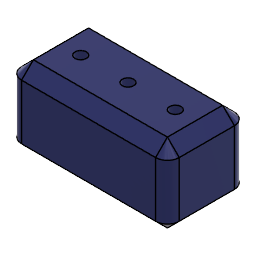
Bed Clamp (Autodesk Fusion 360 design; units mm, degrees)
Autodesk Fusion 360 part; units mm, degrees
sketch "Sketch1" plane through (0, 0, 0) normal (0, 1, 0) x (1, 0, 0)
  line L0 (0, 0) -> (40, 0)
  line L1 (40, 0) -> (40, 20)
  line L2 (40, 20) -> (0, 20)
  line L3 (0, 20) -> (0, 0)
  circle A0 centre (8, 10) radius 2.05
  circle A1 centre (20, 10) radius 2.05
  circle A2 centre (32, 10) radius 2.05
  circle A3 centre (8, 10) radius 2.8 construction
  circle A4 centre (32, 10) radius 2.8 construction
  line L4 (5.2, 8.3834) -> (8, 6.7668)
  line L5 (8, 6.7668) -> (10.8, 8.3834)
  line L6 (10.8, 8.3834) -> (10.8, 11.6166)
  line L7 (10.8, 11.6166) -> (8, 13.2332) construction
  line L8 (8, 13.2332) -> (5.2, 11.6166) construction
  line L9 (5.2, 11.6166) -> (5.2, 8.3834)
  line L10 (29.2, 8.3834) -> (32, 6.7668)
  line L11 (32, 6.7668) -> (34.8, 8.3834)
  line L12 (34.8, 8.3834) -> (34.8, 11.6166)
  line L13 (34.8, 11.6166) -> (32, 13.2332) construction
  line L14 (32, 13.2332) -> (29.2, 11.6166) construction
  line L15 (29.2, 11.6166) -> (29.2, 8.3834)
  line L16 (10.8, 11.6166) -> (10.8, 20)
  line L17 (5.2, 11.6166) -> (5.2, 20)
  line L18 (34.8, 11.6166) -> (34.8, 20)
  line L19 (29.2, 11.6166) -> (29.2, 20)
  circle A5 centre (20, 10) radius 1.45
  circle A6 centre (32, 10) radius 1.45
  circle A7 centre (8, 10) radius 1.45
  line L20 (17.2, 8.3834) -> (20, 6.7668)
  line L21 (20, 6.7668) -> (22.8, 8.3834)
  line L22 (22.8, 8.3834) -> (22.8, 11.6166)
  line L23 (22.8, 11.6166) -> (20, 13.2332) construction
  line L24 (20, 13.2332) -> (17.2, 11.6166) construction
  line L25 (17.2, 11.6166) -> (17.2, 8.3834)
  line L26 (17.2, 11.6166) -> (17.2, 20)
  line L27 (22.8, 11.6166) -> (22.8, 20)
  point P0 (8, 10)
  point P1 (32, 10)
  point P2 (20, 10)
  dimension "ClampWidth" = 20
  dimension "ClampLength" = 40
  dimension "MagnetHoleDia" = 4.1
  dimension "d7" = 10
  dimension "d11" = 8
  dimension "d14" = 24
  dimension "d15" = 0
  dimension "NutCircum" = 5.6
  dimension "d17" = 10
  dimension "d19" = 5.6
  dimension "d20" = 8
  dimension "d21" = 10
  dimension "d22" = 2.9
  dimension "ScrewDia" = 2.9
  dimension "d24" = 2.9
  constraint coincident L0.start L3.end
  constraint horizontal L0
  constraint perpendicular L0 L1
  constraint perpendicular L0 L3
  constraint horizontal L2
  constraint concentric A0 A3
  constraint coincident P0 A0.centre
  constraint coincident P1 A2.centre
  constraint tangent A3 L7
  constraint tangent A4 L14
  constraint vertical L9
  constraint vertical L12
  constraint coincident L2 L16.end
  constraint perpendicular L2 L16
  constraint coincident L2 L17.end
  constraint perpendicular L2 L17
  constraint coincident L2 L18.end
  constraint perpendicular L2 L18
  constraint coincident L2 L19.end
  constraint perpendicular L2 L19
  constraint concentric A1 A5
  constraint concentric A4 A6
  constraint concentric A0 A7
  constraint coincident P2 A1.centre
  constraint coincident L2 L26.end
  constraint perpendicular L2 L26
  constraint coincident L2 L27.end
  constraint perpendicular L2 L27
  constraint equal L6 L22
  constraint equal L16 L27
  measures "ClampWidth" distance of L0.end L1.end
  measures "ClampLength" distance of L0.start L0.end
  measures "MagnetHoleDia" diameter of A0
  measures "d7" distance of L0 P0
  measures "d11" distance of L3 P0
  measures "NutCircum" diameter of A3
  measures "d17" distance of L0 P0
  measures "d19" diameter of A4
  measures "d20" distance of L1 P1
  measures "d21" distance of L0 P1
  measures "d22" diameter of A5
  measures "ScrewDia" diameter of A6
  measures "d24" diameter of A7
extrude "Extrude1" add sketch "Sketch1" along normal blind 20 contours L0 L1 L2 L3 L4 L5 L6 L9 L10 L11 L12 L15 L16 L17 L18 L19 L20 L21 L22 L25 L26 L27 | L2 L4 L5 L6 L9 L16 L17 | L2 L10 L11 L12 L15 L18 L19 | L2 L20 L21 L22 L25 L26 L27 | A0 | A1 | A2 | A5 | A6 | A7
extrude "Extrude2" cut sketch "Sketch1" along normal blind 2.2 contours A0 | A1 | A2 | A5 | A6 | A7
extrude "Extrude3" cut sketch "Sketch1" along normal blind 20 contours A5 | A6 | A7
extrude "Extrude4" cut sketch "Sketch1" against normal blind 2.6 from surface at 15 contours L2 L4 L5 L6 L9 L16 L17 | L2 L10 L11 L12 L15 L18 L19 | L2 L20 L21 L22 L25 L26 L27 | A0 | A1 | A2
fillet "Fillet1" radius 3 4 edges at (40, 10, -20) (40, 10, 0) (0, 10, 0) (0, 10, -20)
chamfer "Chamfer1" distance 3 angle 45 8 edges at (20, 20, -20) (40, 20, -10) (20, 20, 0) (0, 20, -10) (0, 0, -10) (20, 0, -20) (20, 0, 0) (40, 0, -10)
equation "d7 = ClampWidth / 2"
equation "d11 = ClampLength / 5"
equation "d14 = ClampLength * 3 / 5"
equation "d17 = ClampWidth / 2"
equation "d19 = NutCircum"
equation "d20 = ClampLength / 5"
equation "d21 = ClampWidth / 2"
equation "d22 = ScrewDia"
equation "d24 = ScrewDia"
equation "TotalHeight = 20 mm"
equation "d29 = TotalHeight"
equation "NutTopOffset = 5 mm"
equation "NutWidth = 2.6 mm"
equation "d33 = TotalHeight - NutTopOffset"
equation "d34 = -NutWidth"
